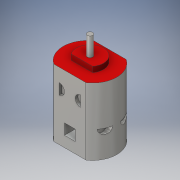
# Autodesk Inventor part: Motor
Saved by Autodesk Inventor 2016 SP2 (Build 200236200, 236)
## iProperties
Created: 2017-06-02
Part Number: Motor
Material: Aluminio 6061-O
Document SubType Name: Modeling
Designer: ssant
Density: 2.7 g/cm^3
Appearance: Aluminio - Pulido
Author: ssant
Autodesk Inventor part; units mm, degrees
ref_plane "XZ Plane" through (0, 0, 0) normal (0, 1, 0) x (-1, 0, 0)
ref_plane "XY Plane" through (0, 0, 0) normal (0, 0, 1) x (1, 0, 0)
sketch "Boceto1" plane through (0, 0, 0) normal (0, 1, 0) x (-1, 0, 0)
  line L0 (10, 7.5) -> (-10, 7.5)
  line L1 (-10, 7.5) -> (-10, -7.5)
  line L2 (-10, -7.5) -> (10, -7.5)
  line L3 (10, -7.5) -> (10, 7.5)
  arc A0 (6, -7.5) -> (6, 7.5) centre (0.9688, 0) ccw
  arc A1 (-6, 7.5) -> (-6, -7.5) centre (-0.9688, 0) ccw
  point P0 (0, 0)
  point P1 (-10, 0)
  point P2 (0, -7.5)
  dimension "d0" = 20
  dimension "d1" = 15
  dimension "d2" = 4
  dimension "d3" = 4
  dimension "d4" = 4
  dimension "d5" = 4
  constraints: 8 end point, 4 point on circle, 4 point on line, 2 centre point, 2 midpoint, 2 parallel, 2 tangent, 1 horizontal, 1 horizontal alignment, 1 perpendicular, 1 vertical alignment
  measures "d0" distance of L2.end L1.end
  measures "d1" distance of L1.end L0.end
  measures "d2" distance of L2.end A0.start
  measures "d3" distance of L0.start A0.end
  measures "d4" distance of L1.end A1.end
  measures "d5" distance of L0.end A1.start
extrude "Extrusión1" add sketch "Boceto1" along normal blind 25 contours A0 L2 A1 L0
sketch "Boceto2" plane through (0, 25, 0) normal (0, 1, 0) x (1, 0, 0)
  line L0 (-6, -7.5) -> (6, -7.5) projected
  arc A0 (6, -7.5) -> (6, 7.5) centre (0.9688, 0) ccw projected
  line L1 (6, 7.5) -> (-6, 7.5) projected
  arc A1 (-6, 7.5) -> (-6, -7.5) centre (-0.9688, 0) ccw projected
  arc A2 (4, -3) -> (-4, -3) centre (0, 0) ccw
  line L2 (0, 0) -> (0, -3)
  line L3 (0, -3) -> (-4, -3)
  line L4 (0, -3) -> (4, -3)
  dimension "d8" = 10
  dimension "d9" = 3
  constraints: 6 end point, 2 point on circle, 1 centre point, 1 coincident, 1 horizontal, 1 point on line, 1 vertical
  measures "d8" diameter of A2
  measures "d9" distance of L2.start L2.end
extrude "Extrusión2" add sketch "Boceto2" along normal blind 2 contours L4 L3 A2
sketch "Boceto3" plane through (0, 27, 0) normal (0, 1, 0) x (1, 0, 0)
  line L0 (-4, -3) -> (4, -3) projected
  arc A0 (4, -3) -> (-4, -3) centre (0, 0) ccw projected
  circle A1 centre (0, 0) radius 1
  dimension "d12" = 2
  constraints: 1 centre point, 1 coincident
  measures "d12" diameter of A1
extrude "Extrusión3" add sketch "Boceto3" along normal blind 7 contours A1
sketch "Boceto4" plane through (-6, 0, 7.5) normal (0, 0, 1) x (1, 0, 0)
  line L0 (0, 0) -> (12, 0) projected
  line L1 (12, 0) -> (12, 25) projected
  line L2 (0, 25) -> (12, 25) projected
  line L3 (0, 0) -> (0, 25) projected
  line L4 (4, 8) -> (8, 8)
  line L5 (8, 8) -> (8, 4)
  line L6 (8, 4) -> (4, 4)
  line L7 (4, 4) -> (4, 8)
  arc A0 (10, 20) -> (10, 16) centre (10, 18) ccw
  line L8 (10, 20) -> (10, 16) construction
  line L9 (10, 20) -> (14, 20) construction
  arc A1 (2, 16) -> (2, 20) centre (2, 18) ccw
  line L10 (2, 20) -> (2, 16) construction
  line L11 (2, 20) -> (6, 20) construction
  line L12 (10, 20) -> (10, 16)
  line L13 (2, 16) -> (2, 20)
  point P0 (6, 0)
  point P1 (6, 4)
  point P2 (6, 0)
  dimension "d15" = 4
  dimension "d16" = 4
  dimension "d17" = 8
  dimension "d18" = 4
  dimension "d19" = 90
  dimension "d20" = 2
  dimension "d21" = 20
  dimension "d22" = 2
  dimension "d23" = 4
  dimension "d24" = 90
  dimension "d25" = 2
  dimension "d26" = 20
  dimension "d27" = 2
  constraints: 20 end point, 4 point on circle, 3 equal length, 3 horizontal, 3 perpendicular, 2 centre point, 2 midpoint, 1 vertical alignment
  measures "d15" distance of L5.end L6.end
  measures "d16" distance of L4.end L5.end
  measures "d17" distance between parallel lines of L0 L4
  measures "d18" distance of L8.start L8.end
  measures "d19" angle of L8 L9
  measures "d20" radius of A0
  measures "d21" distance from line of L0 L8.start
  measures "d22" horizontal distance of L0.end L8.end
  measures "d23" distance of L10.start L10.end
  measures "d24" angle of L10 L11
  measures "d25" radius of A1
  measures "d26" vertical distance of L0.start L10.start
  measures "d27" horizontal distance of L0.start L10.end
extrude "Extrusión4" cut sketch "Boceto4" against normal blind 1 contours L12 A0 | L13 A1
extrude "Extrusión5" cut sketch "Boceto4" against normal blind 8 contours L4 L5 L6 L7
ref_plane "Plano de trabajo1" through (10, 0, 0) normal (1, 0, 0) x (0, 1, 0)
sketch "Boceto5" plane through (10, 0, 0) normal (1, 0, 0) x (0, 1, 0)
  line L0 (0, 7.5) -> (0, -7.5) projected
  line L1 (0, -7.5) -> (25, -7.5) projected
  line L2 (25, 7.5) -> (25, -7.5) projected
  line L3 (0, 7.5) -> (25, 7.5) projected
  arc A0 (10, 5.5) -> (10, 1.5) centre (10, 3.5) ccw
  line L4 (10, 5.5) -> (10, 1.5)
  arc A1 (10, -1.5) -> (10, -5.5) centre (10, -3.5) ccw
  line L5 (10, -5.5) -> (10, -1.5)
  point P0 (0, 0)
  dimension "d32" = 4
  dimension "d33" = 2
  dimension "d34" = 10
  dimension "d35" = 2
  dimension "d36" = 4
  dimension "d37" = 2
  dimension "d38" = 10
  dimension "d39" = 2
  constraints: 4 end point, 4 point on circle, 2 centre point, 2 vertical
  measures "d32" distance of L4.start L4.end
  measures "d33" radius of A0
  measures "d34" distance between parallel lines of L0 L4
  measures "d35" distance from line of L3 L4.start
  measures "d36" distance of L5.end L5.start
  measures "d37" radius of A1
  measures "d38" distance between parallel lines of L0 L5
  measures "d39" vertical distance of L0.end L5.start
extrude "Extrusión6" cut sketch "Boceto5" against normal blind 2 contours L4 A0 | L5 A1
ref_plane "Plano de trabajo2" through (-10, 0, 0) normal (1, 0, 0) x (0, 1, 0)
sketch "Boceto6" plane through (-10, 0, 0) normal (1, 0, 0) x (0, 1, 0)
  line L0 (0, -7.5) -> (0, 7.5) projected
  line L1 (0, 7.5) -> (25, 7.5) projected
  line L2 (25, -7.5) -> (25, 7.5) projected
  line L3 (0, -7.5) -> (25, -7.5) projected
  arc A0 (10, -1.5) -> (10, -5.5) centre (10, -3.5) ccw projected
  line L4 (10, -1.5) -> (10, -5.5) projected
  line L5 (10, -5.5) -> (10, -1.5)
  arc A1 (10, 5.5) -> (10, 1.5) centre (10, 3.5) ccw projected
  line L6 (10, 5.5) -> (10, 1.5) projected
  line L7 (10, 5.5) -> (10, 1.5)
  point P0 (0, 0)
  constraints: 4 end point, 2 collinear
extrude "Extrusión7" cut sketch "Boceto6" along normal blind 2 contours L4 A0 | L6 A1
sketch "Boceto7" plane through (0, 0, 0) normal (0, -1, 0) x (1, 0, 0)
  line L0 (-6, 7.5) -> (6, 7.5) projected
  arc A0 (-6, 7.5) -> (-6, -7.5) centre (-0.9688, 0) ccw projected
  line L1 (6, -7.5) -> (-6, -7.5) projected
  arc A1 (6, -7.5) -> (6, 7.5) centre (0.9688, 0) ccw projected
  circle A2 centre (0, 0) radius 2
  dimension "d44" = 4
  constraints: 1 centre point, 1 coincident
  measures "d44" diameter of A2
extrude "Extrusión8" add sketch "Boceto7" along normal blind 1.75 contours A2
sketch "Boceto8" plane through (0, -1.75, 0) normal (0, -1, 0) x (1, 0, 0)
  circle A0 centre (0, 0) radius 2 projected
  circle A1 centre (0, 0) radius 1
  constraints: 1 centre point, 1 coincident
extrude "Extrusión9" add sketch "Boceto8" along normal blind 0.5 contours A1
